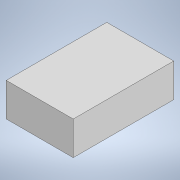
# Autodesk Inventor part: Tunnel
Saved by Autodesk Inventor 2020.4 (Build 244396000, 396)
## iProperties
Created: 2021-04-28
Part Number: Tunnel
Material: Generic
Document SubType Name: Modeling
Designer: armin
Density: 1 g/cm^3
Appearance: Default
Author: armin
Autodesk Inventor part; units mm, degrees
ref_plane "YZ Plane" through (0, 0, 0) normal (1, 0, 0) x (0, 1, 0)
ref_plane "XZ Plane" through (0, 0, 0) normal (0, 1, 0) x (-1, 0, 0)
ref_plane "XY Plane" through (0, 0, 0) normal (0, 0, 1) x (1, 0, 0)
sketch "Sketch1" plane through (0, 0, 0) normal (0, 1, 0) x (-1, 0, 0)
  line L0 (1000, 1500) -> (-1000, 1500)
  line L1 (-1000, 1500) -> (-1000, -1500)
  line L2 (-1000, -1500) -> (1000, -1500)
  line L3 (1000, -1500) -> (1000, 1500)
  line L4 (1000, 1500) -> (-1000, -1500) construction
  line L5 (-1000, 1500) -> (1000, -1500) construction
  point P0 (0, 0)
  dimension "d0" = 2000
  dimension "d1" = 3000
  constraints: 12 end point, 2 midpoint, 2 parallel, 1 horizontal, 1 perpendicular
  measures "d0" distance of L2.end L1.end
  measures "d1" distance of L1.end L0.end
extrude "Extrusion1" add sketch "Sketch1" along normal mid plane 1000
body "Solid1"
